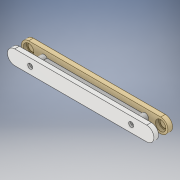
# Autodesk Inventor part: Thigh
Saved by Autodesk Inventor 2019.1 (Build 231200000, 200)
## iProperties
Created: 2018-10-31
Part Number: Thigh
Material: Generisch
Document SubType Name: Modeling
Designer: JochenAlt
Density: 1 g/cm^3
Appearance: Vorgabe
Author: JochenAlt
Autodesk Inventor part; units mm, degrees
ref_plane "YZ Plane" through (0, 0, 0) normal (1, 0, 0) x (0, 1, 0)
ref_plane "XZ Plane" through (0, 0, 0) normal (0, 1, 0) x (-1, 0, 0)
ref_plane "XY Plane" through (0, 0, 0) normal (0, 0, 1) x (1, 0, 0)
sketch "Skizze1" plane through (0, 0, 0) normal (0, 0, 1) x (1, 0, 0)
  circle A0 centre (0, 0) radius 5
  circle A1 centre (127.5, 0) radius 5
  line L0 (0, 7) -> (127.5, 7)
  line L1 (0, -7) -> (127.5, -7)
  line L2 (0, 9.8) -> (0, -9.8) construction
  line L3 (-35.3, 0) -> (162.8, 0) construction
  circle A2 centre (0, 0) radius 7
  circle A3 centre (127.5, 0) radius 7
  circle A4 centre (0, 0) radius 4
  circle A5 centre (127.5, 0) radius 4
  line L4 (17.8267, -1.5) -> (109.6733, -1.5)
  line L5 (112.5, -3) -> (112.5, 0)
  line L6 (109.6733, 1.5) -> (17.8267, 1.5)
  arc A6 (17.8267, 1.5) -> (17.8267, -1.5) centre (15, 0) ccw
  arc A7 (109.6733, -1.5) -> (109.6733, 1.5) centre (112.5, 0) ccw
  circle A8 centre (15, 0) radius 1.2
  circle A9 centre (112.5, 0) radius 1.2
  circle A10 centre (15, 0) radius 2.4
  circle A11 centre (112.5, 0) radius 2.4
  dimension "d0" = 10
  dimension "d2" = 127.5
  dimension "d3" = 2
  dimension "d6" = 1
  dimension "d14" = 15
  dimension "d15" = 3
  dimension "d16" = 3
  dimension "d17" = 15
  dimension "d18" = 2.4
  dimension "d19" = 2
  dimension "d20" = 4.8
  constraints: 12 centre point, 10 end point, 8 coincident, 8 point on circle, 6 equal radius, 4 tangent, 3 point on line, 1 horizontal, 1 parallel, 1 perpendicular, 1 other
  measures "d0" diameter of A0
  measures "d2" distance of A1.centre point (0, 0)
  measures "d3" radial gap between concentric circles of A2 A0
  measures "d6" radial gap between concentric circles of A0 A4
  measures "d14" distance from line of A1.centre L5
  measures "d15" distance of L5.start L5.end
  measures "d16" distance between parallel lines of L4 L6
  measures "d17" distance of A6.centre point (0, 0)
  measures "d18" diameter of A8
  measures "d19" radial gap between concentric circles of A8 A6
  measures "d20" diameter of A10
extrude "Extrusion1" add sketch "Skizze1" along normal blind 7.5 contours L0 A3 L1 A2 | A2 | A3 | A6 L6 A7 L4 | A10 | A11
extrude "Extrusion2" add sketch "Skizze1" along normal blind 0.5 from surface at 7.5 contours A0 | A1 | L0 A3 L1 A2 | A2 | A3 | A6 L6 A7 L4 | A8 | A9 | A10 | A11
extrude "Extrusion3" cut sketch "Skizze1" along normal blind 4.5 contours L0 A3 L1 A2 | A2 | A3 | A6 L6 A7 L4 | A8 | A9 | A10 | A11
extrude "Extrusion4" add sketch "Skizze1" along normal blind 1 from surface at 8 contours A0 | A1 | L0 A3 L1 A2 | A2 | A3 | A4 | A5 | A6 L6 A7 L4 | A10 | A11
extrude "Extrusion5" cut sketch "Skizze1" against normal blind 1.8 from surface at 9 contours A8 | A9 | A10 | A11
mirror "Spiegeln1" about plane through (0, 0, 0) normal (0, 0, 1) bodies 1 separate body
extrude "Extrusion6" add sketch "Skizze1" against normal up to surface (9 mm away) from surface at 4.5 contours A6 L6 A7 L4 | A10 | A11 bodies 1
equation "\"d14\" = d17"
